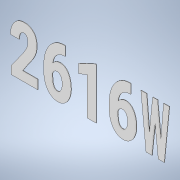
# Autodesk Inventor part: License Plate Numbers
Saved by Autodesk Inventor 2022.2 (Build 262287010, 287A)
## iProperties
Created: 2022-06-18
Part Number: License Plate Numbers
Material: Generic
Document SubType Name: Modeling
Designer: Main Account
Density: 1 g/cm^3
Appearance: Default
Author: Main Account
Autodesk Inventor part; units mm, degrees
ref_plane "YZ Plane" through (0, 0, 0) normal (1, 0, 0) x (0, 1, 0)
ref_plane "XZ Plane" through (0, 0, 0) normal (0, 1, 0) x (-1, 0, 0)
ref_plane "XY Plane" through (0, 0, 0) normal (0, 0, 1) x (1, 0, 0)
sketch "Sketch1" plane through (0, 0, 0) normal (0, 0, 1) x (1, 0, 0)
  line L0 (36, 0) -> (52.5, 0) construction
  line L1 (52.5, 0) -> (52.5, -32) construction
  line L2 (52.5, -32) -> (36, -32) construction
  line L3 (36, -32) -> (36, 0) construction
  line L4 (52.5, -32) -> (54, -32) construction
  line L5 (54, 0) -> (70.5, 0) construction
  line L6 (70.5, 0) -> (70.5, -32) construction
  line L7 (70.5, -32) -> (54, -32) construction
  line L8 (54, -32) -> (54, 0) construction
  line L9 (70.5, -32) -> (72, -32) construction
  line L10 (0, 0) -> (16.5, 0) construction
  line L11 (16.5, 0) -> (16.5, -32) construction
  line L12 (16.5, -32) -> (0, -32) construction
  line L13 (0, -32) -> (0, 0) construction
  line L14 (16.5, -32) -> (18, -32) construction
  line L15 (18, -32) -> (18, 0) construction
  line L16 (18, 0) -> (34.5, 0) construction
  line L17 (34.5, 0) -> (34.5, -32) construction
  line L18 (34.5, -32) -> (18, -32) construction
  line L19 (34.5, -32) -> (36, -32) construction
  line L20 (72, -32) -> (72, 0) construction
  line L21 (72, 0) -> (88.5, 0) construction
  line L22 (88.5, 0) -> (88.5, -32) construction
  line L23 (88.5, -32) -> (72, -32) construction
  circle A0 centre (88.5, -32) radius 0.0013
  circle A1 centre (0, 0) radius 0.0013
  line L24 (15.6093, -30.1658) -> (1.0059, -30.1658)
  line L25 (1.0059, -30.1658) -> (1.0059, -25.9276)
  line L26 (1.0059, -25.9276) -> (7.7317, -16.5067)
  spline S0 degree 2 poles (7.7317, -16.5067) (10.2194, -12.7292) (10.2194, -10.518) knots 0 0 0 1 1 1
  spline S1 degree 2 poles (10.2194, -10.518) (10.2194, -8.7213) (9.0447, -6.8325) (7.916, -6.8325) knots 0 0 0 1 2 2 2
  spline S2 degree 2 poles (7.916, -6.8325) (6.8104, -6.8325) (5.4284, -9.3432) (5.4284, -11.209) knots 0 0 0 1 2 2 2
  line L27 (5.4284, -11.209) -> (0.5682, -11.209)
  spline S3 degree 2 poles (0.5682, -11.209) (0.5682, -8.6522) (2.5031, -4.2988) (5.9121, -1.8342) (8.0312, -1.8342) knots 0 0 0 1 2 3 3 3
  spline S4 degree 2 poles (8.0312, -1.8342) (11.4402, -1.8342) (15.1026, -6.0264) (15.1026, -9.9191) knots 0 0 0 1 2 2 2
  spline S5 degree 2 poles (15.1026, -9.9191) (15.1026, -11.5775) (14.1812, -14.7101) (12.2233, -18.1421) (10.0812, -20.9983) knots 0 0 0 1 2 3 3 3
  line L28 (10.0812, -20.9983) -> (7.3632, -25.1675)
  line L29 (7.3632, -25.1675) -> (15.6093, -25.1675)
  line L30 (15.6093, -25.1675) -> (15.6093, -30.1658)
  line L31 (30.707, -1.6384) -> (30.707, -6.7289)
  line L32 (30.707, -6.7289) -> (30.4997, -6.7289)
  spline S6 degree 2 poles (30.4997, -6.7289) (27.7817, -6.7289) (24.2806, -10.184) (23.866, -13.2705) knots 0 0 0 1 2 2 2
  spline S7 degree 2 poles (23.866, -13.2705) (25.5244, -11.1284) (28.0121, -11.1284) knots 0 0 0 1 1 1
  spline S8 degree 2 poles (28.0121, -11.1284) (30.7301, -11.1284) (33.9548, -16.4261) (33.9548, -20.7334) knots 0 0 0 1 2 2 2
  spline S9 degree 2 poles (33.9548, -20.7334) (33.9548, -23.3823) (32.066, -27.8509) (28.7031, -30.3616) (26.6301, -30.3616) knots 0 0 0 1 2 3 3 3
  spline S10 degree 2 poles (26.6301, -30.3616) (24.4188, -30.3616) (20.8946, -27.6666) (18.9368, -22.6222) (18.9137, -19.3514) knots 0 0 0 1 2 3 3 3
  line L33 (18.9137, -19.3514) -> (18.9137, -16.7486)
  spline S11 degree 2 poles (18.9137, -16.7486) (18.9137, -12.4413) (21.7008, -5.5542) (26.8374, -1.6384) (29.97, -1.6384) knots 0 0 0 1 2 3 3 3
  line L34 (29.97, -1.6384) -> (30.707, -1.6384)
  spline S12 degree 2 poles (26.3306, -16.0806) (25.3632, -16.0806) (24.0733, -17.2784) (23.7508, -18.1306) knots 0 0 0 1 2 2 2
  line L35 (23.7508, -18.1306) -> (23.7508, -20.0655)
  spline S13 degree 2 poles (23.7508, -20.0655) (23.7508, -25.3632) (26.5149, -25.3632) knots 0 0 0 1 1 1
  spline S14 degree 2 poles (26.5149, -25.3632) (27.6205, -25.3632) (29.0947, -22.7144) (29.0947, -20.7104) knots 0 0 0 1 2 2 2
  spline S15 degree 2 poles (29.0947, -20.7104) (29.0947, -18.6604) (27.5975, -16.0806) (26.3306, -16.0806) knots 0 0 0 1 2 2 2
  line L36 (47.7396, -29.97) -> (42.8795, -29.97)
  line L37 (42.8795, -29.97) -> (42.8795, -9.3087)
  line L38 (42.8795, -9.3087) -> (38.1115, -11.1744)
  line L39 (38.1115, -11.1744) -> (38.1115, -6.2682)
  line L40 (38.1115, -6.2682) -> (47.302, -2.03)
  line L41 (47.302, -2.03) -> (47.7396, -2.03)
  line L42 (47.7396, -2.03) -> (47.7396, -29.97)
  line L43 (66.707, -1.6384) -> (66.707, -6.7289)
  line L44 (66.707, -6.7289) -> (66.4997, -6.7289)
  spline S16 degree 2 poles (66.4997, -6.7289) (63.7817, -6.7289) (60.2806, -10.184) (59.866, -13.2705) knots 0 0 0 1 2 2 2
  spline S17 degree 2 poles (59.866, -13.2705) (61.5244, -11.1284) (64.0121, -11.1284) knots 0 0 0 1 1 1
  spline S18 degree 2 poles (64.0121, -11.1284) (66.7301, -11.1284) (69.9548, -16.4261) (69.9548, -20.7334) knots 0 0 0 1 2 2 2
  spline S19 degree 2 poles (69.9548, -20.7334) (69.9548, -23.3823) (68.066, -27.8509) (64.7031, -30.3616) (62.6301, -30.3616) knots 0 0 0 1 2 3 3 3
  spline S20 degree 2 poles (62.6301, -30.3616) (60.4188, -30.3616) (56.8946, -27.6666) (54.9368, -22.6222) (54.9137, -19.3514) knots 0 0 0 1 2 3 3 3
  line L45 (54.9137, -19.3514) -> (54.9137, -16.7486)
  spline S21 degree 2 poles (54.9137, -16.7486) (54.9137, -12.4413) (57.7008, -5.5542) (62.8374, -1.6384) (65.97, -1.6384) knots 0 0 0 1 2 3 3 3
  line L46 (65.97, -1.6384) -> (66.707, -1.6384)
  spline S22 degree 2 poles (62.3306, -16.0806) (61.3632, -16.0806) (60.0733, -17.2784) (59.7508, -18.1306) knots 0 0 0 1 2 2 2
  line L47 (59.7508, -18.1306) -> (59.7508, -20.0655)
  spline S23 degree 2 poles (59.7508, -20.0655) (59.7508, -25.3632) (62.5149, -25.3632) knots 0 0 0 1 1 1
  spline S24 degree 2 poles (62.5149, -25.3632) (63.6205, -25.3632) (65.0947, -22.7144) (65.0947, -20.7104) knots 0 0 0 1 2 2 2
  spline S25 degree 2 poles (65.0947, -20.7104) (65.0947, -18.6604) (63.5975, -16.0806) (62.3306, -16.0806) knots 0 0 0 1 2 2 2
  line L48 (83.3941, -19.5587) -> (84.8913, -2.03)
  line L49 (84.8913, -2.03) -> (88.0239, -2.03)
  line L50 (88.0239, -2.03) -> (85.2368, -29.97)
  line L51 (85.2368, -29.97) -> (81.966, -29.97)
  line L52 (81.966, -29.97) -> (80.2154, -14.0536)
  line L53 (80.2154, -14.0536) -> (78.4879, -29.97)
  line L54 (78.4879, -29.97) -> (75.2171, -29.97)
  line L55 (75.2171, -29.97) -> (72.407, -2.03)
  line L56 (72.407, -2.03) -> (75.5626, -2.03)
  line L57 (75.5626, -2.03) -> (77.0598, -19.5587)
  line L58 (77.0598, -19.5587) -> (78.8795, -2.03)
  line L59 (78.8795, -2.03) -> (81.5514, -2.03)
  line L60 (81.5514, -2.03) -> (83.3941, -19.5587)
  dimension "d4" = 16.5
  dimension "d5" = 1.5
  dimension "d9" = 16.5
  dimension "d10" = 1.5
  dimension "d11" = 32
  dimension "d12" = 16.5
  dimension "d13" = 1.5
  dimension "d15" = 16.5
  dimension "d16" = 1.5
  dimension "d18" = 16.5
  dimension "d26" = 0.0025
  dimension "d28" = 0.0025
  constraints: 8 end point, 7 coincident, 4 horizontal, 2 centre point, 10 other
  measures "d4" distance of L1.end L2.end
  measures "d5" distance of L1.end L4.end
  measures "d9" distance of L6.end L8.start
  measures "d10" distance of L6.end L9.end
  measures "d11" distance of L13.start L13.end
  measures "d12" distance of L11.end L13.start
  measures "d13" distance of L11.end L14.end
  measures "d15" distance of L17.end L15.start
  measures "d16" distance of L17.end L19.end
  measures "d18" distance of L22.end L20.start
  measures "d26" diameter of A0
  measures "d28" diameter of A1
extrude "Extrusion1" add sketch "Sketch1" along normal blind 0.254 contours L24 L25 L26 S0 S1 S2 L27 S3 S4 S5 L28 L29 L30 | L31 L32 S6 S7 S8 S9 S10 L33 S11 L34 | L36 L37 L38 L39 L40 L41 L42 | L43 L44 S16 S17 S18 S19 S20 L45 S21 L46 | L48 L49 L50 L51 L52 L53 L54 L55 L56 L57 L58 L59 L60
extrude "Extrusion2" add sketch "Sketch1" along normal blind 0.127 contours A0 | A1
body "Solid1"
